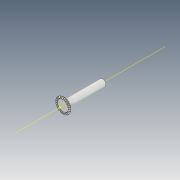
# Autodesk Inventor part: Engrenagem cônica
Saved by Autodesk Inventor 2021 (Build 250183000, 183)
## iProperties
CustomPartVersion: 1
Created: 2020-10-21
Part Number: Engrenagem cônica
Material: Steel, Mild
Document SubType Name: Modeling
Designer: evert
Categories: <?xml version="1.0" encoding="UTF-16"?> <MemberInstance><Categories><FamilyTemplate><FamilyTemplateParameter ValueType="xs:double" Id="1" ObjectReferenceKey="da_z" ObjectType="kUserParameterObject"/><FamilyTemplateParameter ValueType="xs:double" Id="2" ObjectReferenceKey="da_b" ObjectType="kUserParameterObject"/><FamilyTemplateParameter ValueType="xs:double" Id="3" ObjectReferenceKey="da_beta" ObjectType="kUserParameterObject"/><FamilyTemplateParameter ValueType="xs:double" Id="4" ObjectReferenceKey="da_dae" ObjectType="kUserParameterObject"/><FamilyTemplateParameter ValueType="xs:double" Id="5" ObjectReferenceKey="da_ve" ObjectType="kUserParameterObject"/><FamilyTemplateParameter ValueType="xs:double" Id="6" ObjectReferenceKey="da_omega" ObjectType="kUserParameterObject"/><FamilyTemplateParameter ValueType="xs:string" Id="7" ObjectReferenceKey="EAIAABAAAAAAHwAAAAAAAIAAAAAAAAAA" ObjectType="83914240" SubObjectId="SurfaceGeometry"/></FamilyTemplate><ParamToTemplateMap><ParamToTemplate CategoryParameter="//CategoryParameter[@InternalName='046C89C9-8512-4d59-83FE-43B91F4F132A']" TemplateParameter="1"/><ParamToTemplate CategoryParameter="//CategoryParameter[@InternalName='2552DF32-E462-4b46-AEBF-C6C7768E72AC']" TemplateParameter="2"/><ParamToTemplate CategoryParameter="//CategoryParameter[@InternalName='C9EE641D-15FC-4fae-A226-E94C4372FDD7']" TemplateParameter="3"/><ParamToTemplate><ParamToTemplate CategoryParameter="//CategoryParameter[@InternalName='00B6519A-459B-49c7-AD84-2E56D39A5744']" ConstantValue="0.000000"/></ParamToTemplate><ParamToTemplate><ParamToTemplate CategoryParameter="//CategoryParameter[@InternalName='04B31F0E-C7A6-4894-AA32-9629BEFACF47']" ConstantValue="1.000000"/></ParamToTemplate><ParamToTemplate><ParamToTemplate CategoryParameter="//CategoryParameter[@InternalName='43CBEC2E-7847-49e7-A936-2F7889FCB2D9']" ConstantValue="0.200000"/></ParamToTemplate><ParamToTemplate><ParamToTemplate CategoryParameter="//CategoryParameter[@InternalName='B1EFC894-105D-4ebd-86BF-FA20ED196853']" ConstantValue="0.300000"/></ParamToTemplate><ParamToTemplate><ParamToTemplate CategoryParameter="//CategoryParameter[@InternalName='51175063-3D10-4879-93E8-6246FE8B403D']" ConstantValue="2060000000.000000"/></ParamToTemplate><ParamToTemplate><ParamToTemplate CategoryParameter="//CategoryParameter[@InternalName='A3A52E27-4454-46a9-B0BD-C932399B70AF']" ConstantValue="0.300000"/></ParamToTemplate><ParamToTemplate CategoryParameter="//CategoryParameter[@InternalName='2A200944-5A8C-41ca-B96E-8520D2E510F1']" TemplateParameter="4"/><ParamToTemplate><ParamToTemplate CategoryParameter="//CategoryParameter[@InternalName='1A637F62-92C8-44bc-B81F-10802510B579']" ConstantValue="0.378052"/></ParamToTemplate><ParamToTemplate CategoryParameter="//CategoryParameter[@InternalName='B52DD4BE-6863-48fb-BF58-89EF6F9EC65C']" TemplateParameter="5"/><ParamToTemplate><ParamToTemplate CategoryParameter="//CategoryParameter[@InternalName='3956BFF2-84D2-457d-93C2-9B0613DEBA67']" ConstantValue="0.092888"/></ParamToTemplate><ParamToTemplate CategoryParameter="//CategoryParameter[@InternalName='739CFA02-461B-4bf8-8049-181FCAD8B28F']" TemplateParameter="6"/><ParamToTemplate><ParamToTemplate CategoryParameter="//CategoryParameter[@InternalName='A27E999F-E2CE-4481-8A2A-EBF499C4C3C5']" ConstantValue="0.000000"/></ParamToTemplate><ParamToTemplate><ParamToTemplate CategoryParameter="//CategoryParameter[@InternalName='9E1B4470-B2D3-4ff1-B813-535BB4CDF51A']" ConstantValue="3520000.000000"/></ParamToTemplate><ParamToTemplate><ParamToTemplate CategoryParameter="//CategoryParameter[@InternalName='F8452263-BFF6-458c-9FB1-07C4B99E95CD']" ConstantValue="11400000.000000"/></ParamToTemplate><ParamToTemplate><ParamToTemplate CategoryParameter="//CategoryParameter[@InternalName='3E3BB259-FD49-497f-8171-6EBC954A3479']" ConstantValue="2.000000"/></ParamToTemplate><ParamToTemplate CategoryParameter="//CategoryParameter[@InternalName='27C3BAF2-7550-4e4b-AE2C-0DB134B7D9B7']" TemplateParameter="7"/></ParamToTemplateMap><Category DisplayName="Gear" InternalName="DC85795E-93AB-48d5-8EEE-5A27447B64BD" Mnemonic="Gear"><CategoryParameter DisplayName="z" InternalName="046C89C9-8512-4d59-83FE-43B91F4F132A" Mnemonic="z"/><CategoryParameter DisplayName="b" InternalName="2552DF32-E462-4b46-AEBF-C6C7768E72AC" Mnemonic="b"/><CategoryParameter DisplayName="||b|" InternalName="C9EE641D-15FC-4fae-A226-E94C4372FDD7" Mnemonic="beta"/><CategoryParameter DisplayName="x" InternalName="00B6519A-459B-49c7-AD84-2E56D39A5744" Mnemonic="x"/><CategoryParameter DisplayName="a*" InternalName="04B31F0E-C7A6-4894-AA32-9629BEFACF47" Mnemonic="a"/><CategoryParameter DisplayName="c*" InternalName="43CBEC2E-7847-49e7-A936-2F7889FCB2D9" Mnemonic="c"/><CategoryParameter DisplayName="r|.f|*" InternalName="B1EFC894-105D-4ebd-86BF-FA20ED196853" Mnemonic="rf"/><CategoryParameter DisplayName="E" InternalName="51175063-3D10-4879-93E8-6246FE8B403D" Mnemonic="E"/><CategoryParameter DisplayName="||m|" InternalName="A3A52E27-4454-46a9-B0BD-C932399B70AF" Mnemonic="mi"/><Category DisplayName="BevelGear" InternalName="0C98F69A-0C2B-4791-B2FE-7691BB227E77" Mnemonic="BevelGear"><CategoryParameter DisplayName="d|.ae|" InternalName="2A200944-5A8C-41ca-B96E-8520D2E510F1" Mnemonic="dae"/><CategoryParameter DisplayName="d|.ai|" InternalName="1A637F62-92C8-44bc-B81F-10802510B579" Mnemonic="dai"/><CategoryParameter DisplayName="A|.e|" InternalName="B52DD4BE-6863-48fb-BF58-89EF6F9EC65C" Mnemonic="ve"/><CategoryParameter DisplayName="A|.i|" InternalName="3956BFF2-84D2-457d-93C2-9B0613DEBA67" Mnemonic="vi"/><CategoryParameter DisplayName="||S|" InternalName="739CFA02-461B-4bf8-8049-181FCAD8B28F" Mnemonic="omega"/><CategoryParameter DisplayName="x|.t|" InternalName="A27E999F-E2CE-4481-8A2A-EBF499C4C3C5" Mnemonic="xt"/><CategoryParameter DisplayName="||s||.Flim|" InternalName="9E1B4470-B2D3-4ff1-B813-535BB4CDF51A" Mnemonic="sFlim"/><CategoryParameter DisplayName="||s||.Hlim|" InternalName="F8452263-BFF6-458c-9FB1-07C4B99E95CD" Mnemonic="sHlim"/><CategoryParameter DisplayName="tipo" InternalName="3E3BB259-FD49-497f-8171-6EBC954A3479" Mnemonic="type"/><CategoryParameter DisplayName="PitchDiameter" InternalName="27C3BAF2-7550-4e4b-AE2C-0DB134B7D9B7" Mnemonic="IDS_PITCHDIAM"/></Category></Category></Categories></MemberInstance>
Mass: 60.9118 g
Surface Area: 34.3074 cm^2
Volume: 7.7496 cm^3
Density: 7.86 g/cm^3
Appearance: Steel
Author: evert
Autodesk Inventor part; units mm, degrees
ref_plane "Plano de malha 2" through (0, 0, 0) normal (0.9927089, 0.1205367, 0) x (0, 0, 1)
sketch "Esboço de corpo dentado" plane through (0, 0, 0) normal (1, 0, 0) x (0, 1, 0)
  line L0 (0, 0) -> (2.23206, -1.537096) construction
  line L1 (2.23206, -1.537096) -> (2.42995, -1.194087)
  line L2 (2.42995, -1.194087) -> (0, 0) construction
  line L3 (2.34, -1.35) -> (0, 0) construction
  line L4 (1.736322, -1.195709) -> (1.890261, -0.928881)
  line L5 (2.23206, -1.537096) -> (1.736322, -1.195709)
  line L6 (2.42995, -1.194087) -> (1.890261, -0.928881)
  line L7 (0, -39.386751) -> (0, 6.564458)
  line L8 (0, -1.35) -> (2.42995, -1.35) construction
  dimension "d0" = 4.68
  dimension "d1" = 4.46412
  dimension "d2" = 4.8599
  dimension "d3" = 0.6
  dimension "d4" = 1.19409
  constraints: 16 end point, 4 point on line, 3 perpendicular, 2 collinear, 1 horizontal alignment, 1 vertical alignment
  measures "d0" diameter of L3.start L7
  measures "d1" diameter of L0.end L7
  measures "d2" diameter of L1.end L7
  measures "d3" distance between parallel lines of L1 L4
  measures "d4" vertical distance of L1.end L0.start
revolve "Corpo dentado" add sketch "Esboço de corpo dentado" angle 360 about axis through (0, 0, 0) along (0, 0, 1)
ref_plane "Plano de dente" through (0, 2.34, -1.35) normal (0, -0.8661856, 0.4997225) x (1, 0, 0)
sketch "Esboço inicial" plane through (0, 2.34, -1.35) normal (0, -0.8661856, 0.4997225) x (1, 0, 0)
  line L0 (0, -23.505131) -> (0, 10.644758)
  arc A0 (-0.064243, -0.26352) -> (-0.292703, 0.290193) centre (-1.691227, -0.61082) ccw
  arc A1 (0.292703, 0.290193) -> (0.064243, -0.26352) centre (1.691227, -0.61082) ccw
  line L1 (-0.064243, -0.26352) -> (0.064243, -0.26352)
  arc A2 (0.292703, 0.290193) -> (-0.292703, 0.290193) centre (0, -4.682599) ccw
  dimension "d7" = 1.66364
  dimension "d8" = 1.69123
  dimension "d9" = 4.07178
  dimension "d57" = 4.9814
  dimension "d58" = 4.41908
  constraints: 6 point on circle, 3 centre point, 3 symmetric about line, 2 end point, 1 coincident, 1 perpendicular, 1 other
  measures "d7" radius of A0
  measures "d8" horizontal distance of point (0, -4.683) A0.centre
  measures "d9" vertical distance of point (0, -4.683) A0.centre
  measures "d57" radius of A2
  measures "d58" distance from line of A2.centre L1
ref_plane "Plano final" through (0, 1.803138, -1.040272) normal (0, -0.8661856, 0.4997225) x (1, 0, 0)
sketch "Esboço final" plane through (0, 1.803138, -1.040272) normal (0, -0.8661856, 0.4997225) x (1, 0, 0)
  line L0 (0, -15.35404) -> (0, 6.953444)
  arc A0 (-0.049504, -0.203061) -> (-0.225548, 0.223615) centre (-1.303212, -0.470681) ccw
  arc A1 (0.225548, 0.223615) -> (0.049504, -0.203061) centre (1.303212, -0.470681) ccw
  line L1 (-0.049504, -0.203061) -> (0.049504, -0.203061)
  arc A2 (0.225548, 0.223615) -> (-0.225548, 0.223615) centre (0, -3.608279) ccw
  dimension "d12" = 1.28195
  dimension "d15" = 1.30321
  dimension "d16" = 3.1376
  dimension "d59" = 3.83853
  dimension "d60" = 3.40522
  constraints: 6 point on circle, 3 centre point, 3 symmetric about line, 2 end point, 1 coincident, 1 other
  measures "d12" radius of A0
  measures "d15" horizontal distance of A0.centre point (0, -3.608)
  measures "d16" vertical distance of A0.centre point (0, -3.608)
  measures "d59" radius of A2
  measures "d60" distance from line of A2.centre L1
loft "Loft" cut profiles "Esboço inicial", "Esboço final"
pattern_circular "Circular Pattern" count 26 over 360 about axis through (0, 0, 0) along (0, 0, 1) of "Loft"
sketch3d "Esboço 3D direito"
ref_plane "Plano final direito" through (-0.195165, 1.792545, -1.040272) normal (0.0937526, -0.8610969, 0.4997225) x (0.9941252, 0.1082362, 0)
sketch "Esboço final direita" plane through (-0.195165, 1.792545, -1.040272) normal (0.0937526, -0.8610969, 0.4997225) x (0.9941252, 0.1082362, 0)
  arc A0 (-0.049504, -0.203061) -> (-0.225548, 0.223615) centre (-1.303212, -0.470681) ccw
  line L0 (0, -16.345992) -> (0, 7.945385)
  arc A1 (0.225548, 0.223615) -> (0.049504, -0.203061) centre (1.303212, -0.470681) ccw
  line L1 (-0.049504, -0.203061) -> (0.049504, -0.203061)
  arc A2 (0.225548, 0.223615) -> (-0.225548, 0.223615) centre (0, -3.608279) ccw
  dimension "d70" = 1.30321
  dimension "d71" = 3.1376
  dimension "d72" = 1.28195
  dimension "d73" = 3.40522
  dimension "d74" = 3.83853
  constraints: 6 point on circle, 3 centre point, 3 symmetric about line, 2 end point, 1 coincident, 1 perpendicular, 1 other
  measures "d70" horizontal distance of A2.centre A0.centre
  measures "d71" vertical distance of point (0, -3.608) A0.centre
  measures "d72" radius of A0
  measures "d73" distance from line of point (0, -3.608) L1
  measures "d74" radius of A2
feature "Transição direita" [suppressed]
pattern_circular "Padrão circular direito" [suppressed]
sketch3d "Esboço 3D esquerdo"
ref_plane "Plano final esquerdo" through (0.20202, 1.792545, -1.044699) normal (-0.096912, -0.8599118, 0.5011584) x (0.9937092, -0.111991, 0)
sketch "Esboço final esquerdo" plane through (0.20202, 1.792545, -1.044699) normal (-0.096912, -0.8599118, 0.5011584) x (0.9937092, -0.111991, 0)
  line L0 (0, -27.757202) -> (0, 10.734479)
  arc A0 (-0.049504, -0.199604) -> (-0.225548, 0.227072) centre (-1.303212, -0.467223) ccw
  arc A1 (0.225548, 0.227072) -> (0.049504, -0.199604) centre (1.303212, -0.467223) ccw
  line L1 (-0.049504, -0.199604) -> (0.049504, -0.199604)
  ellipse E0 centre (0, -0.803813) end of major axis (1.890261, -0.803813) minor radius 0.94732
  arc A2 (0.225548, 0.227072) -> (-0.225548, 0.227072) centre (0, -3.604822) ccw
  dimension "d56" = 0.94732
  dimension "d30" = 1.28195
  dimension "d31" = 1.30321
  dimension "d32" = 3.1376
  dimension "d61" = 3.83853
  dimension "d62" = 3.40522
  constraints: 6 point on circle, 3 centre point, 3 symmetric about line, 2 end point, 1 coincident, 2 other
  measures "d30" radius of A0
  measures "d31" horizontal distance of point (0, -3.605) A0.centre
  measures "d32" vertical distance of A0.centre point (0, -3.605)
  measures "d61" radius of A2
  measures "d62" distance from line of point (0, -3.605) L1
feature "Transição esquerda" [suppressed]
pattern_circular "Padrão circular esquerdo" [suppressed]
sketch "Esboço de corpo" plane through (0, 0, 0) normal (1, 0, 0) x (0, 1, 0)
  line L0 (0, -35.037536) -> (0, -19.530831)
  line L1 (2.23206, -1.537096) -> (1.736322, -1.195709)
  line L2 (1.736322, -1.195709) -> (0, -1.195709)
  line L3 (2.23206, -1.537096) -> (0, -1.537096)
  constraints: 4 end point, 2 perpendicular, 2 point on line
sketch "Esboço de corpo outline for Fixar corpo" plane through (0, 0, 0) normal (1, 0, 0) x (0, 1, 0)
  line L0 (0, -1.537096) -> (2.23206, -1.537096)
  line L1 (0, -1.195709) -> (0, -1.537096)
  line L2 (1.736322, -1.195709) -> (0, -1.195709)
  line L3 (2.23206, -1.537096) -> (1.736322, -1.195709)
revolve "Fixar corpo" add sketch "Esboço de corpo outline for Fixar corpo" angle 360 about axis through (0, 0, 0) along (0, 0, 1)
sketch "Sketch6" plane through (0, 0, 0) normal (1, 0, 0) x (0, 1, 0)
  line L0 (2.34, -1.35) -> (0, 0)
  line L1 (0, -37.799919) -> (0, 6.299986)
surface revolve "Diâmetro do flanco" sketch "Sketch6" angle 360 about axis through (0, 0, 0) along (0, 0, 1) shown no curves L0
sketch "Esboço8" plane through (0, 0, -1.537096) normal (0, 0, -1) x (-1, 0, 0)
  circle A0 centre (0, 0) radius 1
  constraints: 1 centre point, 1 coincident
extrude "Extrusão1" add sketch "Esboço8" along normal blind 12.5
equation "\"d0\" = da_de"
equation "\"d1\" = da_dfe"
equation "\"d2\" = da_dae"
equation "\"d3\" = da_b"
equation "\"d4\" = da_ve"
equation "\"d7\" = fd_rr"
equation "\"d8\" = fd_x"
equation "\"d9\" = fd_y"
equation "\"d57\" = 0.5 * fd_dva + 0.3 * da_he"
equation "\"d58\" = 0.5 * fd_dva - 1.12 * da_he"
equation "\"da_teethtype\" = 0"
equation "\"da_b\" = 0.6"
equation "\"da_de\" = 4.68"
equation "\"da_dae\" = 4.8599"
equation "\"da_dfe\" = 4.46412"
equation "\"da_le\" = 2.7015"
equation "\"da_omega\" = 90deg"
equation "\"da_beta\" = 0"
equation "\"da_delta\" = 60.018361deg"
equation "\"da_alpha\" = 20deg"
equation "\"da_he\" = 0.396"
equation "\"da_ve\" = 1.19409"
equation "\"da_zv\" = 52.028881"
equation "\"fd_loft\" = da_b + 0.05 * da_he"
equation "\"fd_x\" = fd_x1 + fd_x2"
equation "\"fd_y\" = fd_y1 - fd_y2"
equation "\"fd_dd\" = fd_dva - 0.8 * da_he"
equation "\"da_dvw\" = 9.3652"
equation "\"d11\" = fd_loft"
equation "\"da_dm\" = 4.16029"
equation "\"da_x\" = 0"
equation "\"da_m\" = 0.18"
equation "\"d50\" = da_omega"
equation "\"fd_rr\" = 1.663639"
equation "\"fd_dva\" = 9.725199"
equation "\"fd_x1\" = 0.14292"
equation "\"fd_x2\" = 1.548307"
equation "\"fd_y1\" = 4.680418"
equation "\"fd_y2\" = 0.608638"
body "Solid1"
body "Srf1"
